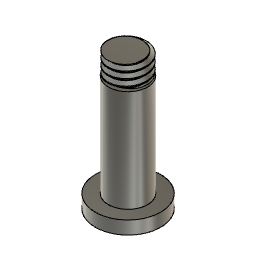
axle wheel rotate (Autodesk Fusion 360 design; units mm, degrees)
Autodesk Fusion 360 part; units mm, degrees
mesh "Mesh1" [no effect] in component "axle wheel rotate"
sketch "axle wheel rotate" plane through (0, 0, 0) normal (0, 0, 1) x (1, 0, 0) in component "axle wheel rotate"
  circle A0 centre (-0.0002, 0.0002) radius 4.9998
  circle A1 centre (-0.0002, 0.0002) radius 3.001
  constraint concentric A0 A1
extrude "Extrude1" add sketch "axle wheel rotate" along normal blind 2 contours A0 | A1 makes body 1 in component "axle wheel rotate"
extrude "Extrude2" add sketch "axle wheel rotate" along normal blind 17.58 contours A1 bodies 1 in component "axle wheel rotate"
extrude "Extrude3" add 1 faces at (-1.2476, 0.2983, 17.58) along direction (0, 0, 1) blind 3.4 separate body on bodies 1 makes body 2 in component "axle wheel rotate"
thread "Thread1" "ISO Metric profile 6.0 M6x1 6g" major diameter 5.884 minor diameter 4.7435 pitch 1 angle 60 modelled right hand crest width 0.1444 on face at (2.9859, -0.2986, 18.7133) crest through (2.9418, 0.0002, 17.33) on bodies 2 in component "axle wheel rotate"
combine "Combine1" operation add target body 1 tool bodies 2 in component "axle wheel rotate"
component "axle wheel rotate" placed x (1, 0, 0) y (0, 1, 0) z (0, 0, 1) at (0, 0, 0)
named bodies: "axle wheel rotate"
